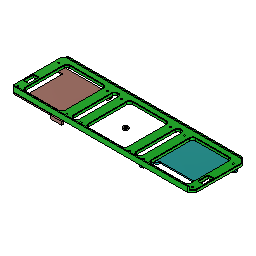
LCD sled v8 (Autodesk Fusion 360 design; units mm, degrees)
Autodesk Fusion 360 part; units mm, degrees
note: some values were not read from the file. Set by a fixed rule: which sketch regions a step uses; the direction of a hole.
sketch "Esquisse1" plane through (0, 0, 0) normal (0, 0, 1) x (1, 0, 0)
  circle A0 centre (107.25, 0) radius 1.25
  line L0 (136, 89.05) -> (136, -3.55)
  line L1 (136, -3.55) -> (-121, -3.55)
  line L2 (-121, -3.55) -> (-121, 89.05)
  line L3 (-121, 89.05) -> (136, 89.05)
  line L4 (108.5, 10.5227) -> (108.5, -1.25) construction
  line L5 (-112.6, 59.85) -> (117.25, 59.85)
  line L6 (117.25, 59.85) -> (117.25, -4.15)
  line L7 (117.25, -4.15) -> (-112.6, -4.15)
  line L8 (-112.6, -4.15) -> (-112.6, 59.85)
  line L9 (108.5, -1.25) -> (-108.5, -1.25) construction
  line L10 (-108.5, -1.25) -> (-108.5, 4.7567) construction
  circle A1 centre (-107.25, 0) radius 1.25
  circle A2 centre (-47.25, 0) radius 1.25
  circle A3 centre (-30, 0) radius 1.25
  circle A4 centre (30, 0) radius 1.25
  circle A5 centre (47.25, 0) radius 1.25
  point P0 (-107.25, 50)
  point P1 (-47.25, 50)
  point P2 (-30, 50)
  point P3 (30, 50)
  point P4 (47.25, 50)
  point P5 (107.25, 50)
  dimension "d1" = 27.5
  dimension "d2" = 8.75
  dimension "d3" = 2.5
  dimension "d4" = 12.5
  dimension "d5" = 5.35
  dimension "d6" = 0.6
  dimension "d7" = 2.3
  dimension "d8" = 60
  dimension "d9" = 60
  dimension "d10" = 60
  dimension "d11" = 17.25
  dimension "d12" = 17.25
  dimension "d13" = 30
  dimension "d14" = 92.6
  dimension "d15" = 64
  dimension "d16" = 50
  constraint vertical L0
  constraint perpendicular L0 L1
  constraint perpendicular L1 L2
  constraint horizontal L3
  constraint vertical L4
  constraint horizontal L5
  constraint vertical L6
  constraint horizontal L7
  constraint vertical L8
  constraint tangent A0 L4
  constraint perpendicular L8 L9
  constraint perpendicular L9 L10
  constraint equal A0 A1
  constraint horizontal origin A0.centre
  constraint horizontal origin A1.centre
  constraint tangent A0 L9
  constraint tangent L10 A1
  constraint equal A1 A2
  constraint tangent L9 A2
  constraint equal A4 A5
  constraint equal A3 A4
  constraint equal A2 A3
  constraint tangent L9 A3
  constraint tangent L9 A4
  constraint tangent L9 A5
  constraint horizontal P4 P5
  constraint horizontal P3 P4
  constraint horizontal P1 P2
  constraint horizontal P0 P1
  constraint vertical A1.centre P0
  constraint vertical A2.centre P1
  constraint vertical A3.centre P2
  constraint vertical A5.centre P4
  constraint vertical A0.centre P5
  constraint vertical A4.centre P3
  constraint horizontal P2 P3
  measures "d1" distance of L0 L4
  measures "d2" distance of L4 L6
  measures "d3" diameter of A0
  measures "d4" distance of L2 L10
  measures "d5" distance of L8 A1.centre
  measures "d6" distance of L1 L7
  measures "d7" distance of L1 L9
  measures "d8" distance of A1.centre A2.centre
  measures "d9" distance of A3.centre A4.centre
  measures "d10" horizontal distance of A0.centre A5.centre
  measures "d11" distance of A4.centre A5.centre
  measures "d12" distance of A2.centre A3.centre
  measures "d13" distance of origin A4.centre
  measures "d14" distance of L0.start L0.end
  measures "d15" distance of L5.end L6.end
  measures "d16" vertical distance of A1.centre P0
ref_plane "Plan de construction1" through (0, 0, 10.5) normal (0, 0, 1) x (1, 0, 0)
sketch "Esquisse2" plane through (0, 0, 10.5) normal (0, 0, 1) x (1, 0, 0)
  line L0 (-112.6, 59.85) -> (117.25, 59.85)
  line L1 (117.25, 59.85) -> (117.25, -4.15)
  line L2 (117.25, -4.15) -> (-112.6, -4.15)
  line L3 (-112.6, -4.15) -> (-112.6, 59.85)
extrude "Extrusion1" add sketch "Esquisse2" against normal blind 6.5 makes body 1
sketch "Esquisse3" plane through (0, 0, 0) normal (1, 0, 0) x (0, 1, 0)
  line L0 (-4.15, 10.5) -> (59.85, 10.5)
  line L1 (59.85, 10.5) -> (59.85, 4)
  line L2 (59.85, 4) -> (-4.15, 4)
  line L3 (-4.15, 4) -> (-4.15, 10.5)
  line L4 (-4.35, 10.7) -> (60.05, 10.7)
  line L5 (60.05, 10.7) -> (60.05, 3.8)
  line L6 (60.05, 3.8) -> (-4.35, 3.8)
  line L7 (-4.35, 3.8) -> (-4.35, 10.7)
  line L8 (-4.35, 6.8) -> (-5.55, 6.8)
  line L9 (-5.55, 6.8) -> (-5.55, 0)
  line L10 (-5.55, 0) -> (61.25, 0)
  line L11 (61.25, 0) -> (61.25, 5.05)
  line L12 (61.25, 5.05) -> (60.05, 5.05)
  dimension "d20" = -0.2
  dimension "d21" = 1.2
  dimension "d22" = 1.2
  dimension "d61" = 3
  dimension "d62" = 1.25
  constraint perpendicular L7 L8
  constraint perpendicular L8 L9
  constraint perpendicular L9 L10
  constraint perpendicular L8 L11
  constraint perpendicular L5 L12
  constraint coincident L10 origin
  constraint coincident L5 L12.end
  constraint coincident L7 L8.start
  measures "d21" distance of L5 L11
  measures "d22" distance of L7 L9
  measures "d61" distance of L6 L8
  measures "d62" vertical distance of L5.end L11.end
extrude "Extrusion2" add sketch "Esquisse3" along normal mid plane 224 separate body contours L5 L6 L7 L8 L9 L10 L11 L12 makes body 2
hole "Perçage1" at (-107.25, 0, 0) at (-47.25, 0, 0) at (-30, 0, 0) at (-30, 50, 0) at (-47.25, 50, 0) at (-107.25, 50, 0) at (30, 50, 0) at (30, 0, 0) at (47.25, 0, 0) at (47.25, 50, 0) at (107.25, 50, 0) at (107.25, 0, 0) direction (0, 0, 1) diameter 2 depth 5 tip angle 180 countersink diameter 2.4 countersink angle 90 bodies 2
sketch "Esquisse4" plane through (0, 0, 0) normal (0, 0, -1) x (1, 0, 0)
  circle A0 centre (107.25, -50) radius 1.2
  circle A1 centre (47.25, 0) radius 1.2
  circle A2 centre (30, -50) radius 1.2
  circle A3 centre (-47.25, -50) radius 1.2
  circle A4 centre (-30, 0) radius 1.2
  circle A5 centre (-107.25, 0) radius 1.2
  circle A6 centre (-47.25, 0) radius 1.2
  circle A7 centre (-30, -50) radius 1.2
  circle A8 centre (-107.25, -50) radius 1.2
  circle A9 centre (30, 0) radius 1.2
  circle A10 centre (47.25, -50) radius 1.2
  circle A11 centre (107.25, 0) radius 1.2
  line L0 (-112, -61.25) -> (112, -61.25)
  line L1 (112, -61.25) -> (112, 5.55)
  line L2 (112, 5.55) -> (-112, 5.55)
  line L3 (-112, 5.55) -> (-112, -61.25)
  line L4 (-110.25, -10) -> (-104.25, -10)
  line L5 (-104.25, -10) -> (-104.25, -22)
  line L6 (-104.25, -22) -> (-110.25, -22)
  line L7 (-110.25, -22) -> (-110.25, -10)
  line L8 (117.25, 4.15) -> (-112.6, 4.15)
  line L9 (-107.25, 0) -> (-107.25, -10) construction
  line L10 (-3, -22) -> (3, -22)
  line L11 (3, -22) -> (3, -10)
  line L12 (3, -10) -> (-3, -10)
  line L13 (-3, -10) -> (-3, -22)
  line L14 (0, 0) -> (0, -10) construction
  line L15 (104.25, -22) -> (110.25, -22)
  line L16 (110.25, -22) -> (110.25, -10)
  line L17 (110.25, -10) -> (104.25, -10)
  line L18 (104.25, -10) -> (104.25, -22)
  line L19 (107.25, 0) -> (107.25, -10) construction
  dimension "d32" = 6
  dimension "d33" = 12
  dimension "d63" = 10
  constraint horizontal L4
  constraint vertical L5
  constraint horizontal L6
  constraint vertical L7
  constraint coincident A5.centre L9.start
  constraint midpoint L4 L9.end
  constraint vertical L9
  constraint horizontal L10
  constraint vertical L11
  constraint horizontal L12
  constraint vertical L13
  constraint coincident L14.start origin
  constraint midpoint L12 L14.end
  constraint vertical L14
  constraint collinear L6 L10
  constraint collinear L4 L12
  constraint equal L6 L10
  constraint horizontal L15
  constraint vertical L16
  constraint horizontal L17
  constraint vertical L18
  constraint coincident A11.centre L19.start
  constraint midpoint L17 L19.end
  constraint vertical L19
  constraint equal L10 L15
  constraint collinear L10 L15
  constraint collinear L12 L17
  measures "d32" distance of L4.start L4.end
  measures "d33" distance of L4.end L5.end
  measures "d63" distance of L4 A5.centre
extrude "Extrusion3" cut sketch "Esquisse4" against normal up to surface (3.8 mm away) contours L4 L5 L6 L7 | L10 L11 L12 L13 | L15 L16 L17 L18 bodies 2
ref_plane "Plan de construction2" through (0, 27.85, -1.6) normal (0, 0, -1) x (0, 1, 0)
sketch "Esquisse5" plane through (0, 27.05, -1.6) normal (0, 0, -1) x (1, 0, 0)
  circle A0 centre (47.25, -22.95) radius 1.5
  circle A1 centre (47.25, 16.55) radius 1
  circle A2 centre (97.25, -22.95) radius 1
  circle A3 centre (107.25, -22.95) radius 1.5
  circle A4 centre (47.25, 27.05) radius 1.5
  line L0 (99.75, -25.7) -> (44.75, -25.7)
  line L1 (44.75, -25.7) -> (44.75, 19.3)
  line L2 (44.75, 19.3) -> (99.75, 19.3)
  line L3 (99.75, 19.3) -> (99.75, -25.7)
  line L4 (107.25, -20.2) -> (97.25, -20.2)
  arc A5 (97.25, -20.2) -> (97.25, -25.7) centre (97.25, -22.95) ccw
  line L5 (97.25, -25.7) -> (107.25, -25.7)
  arc A6 (107.25, -25.7) -> (107.25, -20.2) centre (107.25, -22.95) ccw
  line L6 (107.25, -22.95) -> (97.25, -22.95) construction
  line L7 (44.75, 27.05) -> (44.75, 16.55)
  arc A7 (44.75, 16.55) -> (49.75, 16.55) centre (47.25, 16.55) ccw
  line L8 (49.75, 16.55) -> (49.75, 27.05)
  arc A8 (49.75, 27.05) -> (44.75, 27.05) centre (47.25, 27.05) ccw
  line L9 (47.25, 27.05) -> (47.25, 16.55) construction
  circle A9 centre (47.25, 16.55) radius 2.5
  circle A10 centre (97.25, -22.95) radius 2.5
  circle A11 centre (47.25, -22.95) radius 2.5
  circle A12 centre (97.25, 16.55) radius 2.5
  point P0 (47.25, -22.95)
  point P1 (47.25, 27.05)
  point P2 (107.25, -22.95)
  dimension "d42" = 3
  dimension "d43" = 50
  dimension "d44" = 39.5
  dimension "d45" = 2
  dimension "d46" = 55
  dimension "d48" = 45
  dimension "d49" = 2.75
  dimension "d50" = 2.5
  dimension "d51" = 2.75
  dimension "d52" = 2.5
  constraint coincident P0 A0.centre
  constraint coincident P1 A4.centre
  constraint coincident P2 A3.centre
  constraint equal A0 A3
  constraint equal A3 A4
  constraint equal A1 A2
  constraint horizontal L0
  constraint vertical L1
  constraint horizontal L2
  constraint vertical L3
  constraint vertical A1.centre P1
  constraint horizontal A2.centre P0
  constraint tangent L4 A5
  constraint tangent A5 L5
  constraint parallel L4 L5
  constraint tangent L5 A6
  constraint tangent L4 A6
  constraint coincident A2.centre A5.centre
  constraint horizontal L6
  constraint tangent L7 A7
  constraint tangent A7 L8
  constraint parallel L7 L8
  constraint tangent L8 A8
  constraint tangent L7 A8
  constraint coincident A1.centre A7.centre
  constraint perpendicular L2 L9
  constraint concentric A1 A9
  constraint equal A8 A9
  constraint concentric A5 A10
  constraint tangent L3 A10
  constraint equal A10 A11
  constraint equal A9 A12
  constraint horizontal A1.centre A12.centre
  constraint vertical A2.centre A12.centre
  measures "d42" diameter of A0
  measures "d43" horizontal distance of A2.centre P0
  measures "d44" vertical distance of A1.centre P0
  measures "d45" diameter of A2
  measures "d46" distance of L0.start L0.end
  measures "d48" distance of L0.end L1.end
  measures "d49" distance of A1.centre L2
  measures "d50" distance of A2.centre L3
  measures "d51" radius of A6
  measures "d52" radius of A8
extrude "Extrusion4" add sketch "Esquisse5" along normal blind 2 separate body contours A10 | L0 L3 L4 A5 L5 | L3 L4 L5 A6 | A12 | A11 | L0 L1 L2 L3 L4 A5 A7 L8 A9 | A7 A9 | L1 L2 L7 L8 A9 | L2 L7 L8 A8 makes body 3
extrude "Extrusion5" add sketch "Esquisse5" along normal blind 2 from surface at 2 contours A10 | A12 | A11 | A7 A9 bodies 3
fillet "Congé1" radius 2 4 edges at (99.75, 47.25, -2.6) (99.75, 7.75, -2.6) (49.75, 7.75, -2.6) (44.75, 52.75, -2.6) on bodies 3
chamfer "Chanfrein1" distance 0.5 angle 45 5 edges at (96.3177, 49.6384, -5.6) (46.3177, 10.1384, -5.6) (45.8515, 49.4576, -5.6) (45.8515, -0.5424, -3.6) (105.8515, 49.4576, -3.6) on bodies 3
sketch "Esquisse6" plane through (0, 0, 3.8) normal (0, 0, 1) x (-1, 0, 0)
  line L0 (110.25, -10) -> (110.25, -22)
  line L1 (110.25, -22) -> (104.25, -22)
  line L2 (104.25, -22) -> (104.25, -10)
  line L3 (104.25, -10) -> (110.25, -10)
  line L4 (-3, -10) -> (3, -10)
  line L5 (3, -10) -> (3, -22)
  line L6 (3, -22) -> (-3, -22)
  line L7 (-3, -22) -> (-3, -10)
  line L8 (-110.25, -10) -> (-104.25, -10)
  line L9 (-104.25, -10) -> (-104.25, -22)
  line L10 (-104.25, -22) -> (-110.25, -22)
  line L11 (-110.25, -22) -> (-110.25, -10)
  circle A0 centre (-107.25, -50) radius 1
  circle A1 centre (-47.25, 0) radius 1
  circle A2 centre (-30, -50) radius 1
  circle A3 centre (47.25, -50) radius 1
  circle A4 centre (30, 0) radius 1
  circle A5 centre (107.25, 0) radius 1
  circle A6 centre (47.25, 0) radius 1
  circle A7 centre (30, -50) radius 1
  circle A8 centre (107.25, -50) radius 1
  circle A9 centre (-30, 0) radius 1
  circle A10 centre (-47.25, -50) radius 1
  circle A11 centre (-107.25, 0) radius 1
  line L12 (112, 4.35) -> (-112, 4.35)
  line L13 (-112, 4.35) -> (-112, -60.05)
  line L14 (-112, -60.05) -> (112, -60.05)
  line L15 (112, -60.05) -> (112, 4.35)
  line L16 (101.25, -54.05) -> (53.25, -54.05)
  line L17 (53.25, -54.05) -> (53.25, 0)
  line L18 (53.25, 0) -> (101.25, 0)
  line L19 (101.25, 0) -> (101.25, -54.05)
  line L20 (42.25, -54.05) -> (35, -54.05)
  line L21 (35, -54.05) -> (35, 0)
  line L22 (35, 0) -> (42.25, 0)
  line L23 (42.25, 0) -> (42.25, -54.05)
  line L24 (24, -54.05) -> (-24, -54.05)
  line L25 (-24, -54.05) -> (-24, 0)
  line L26 (-24, 0) -> (24, 0)
  line L27 (24, 0) -> (24, -54.05)
  line L28 (-53.25, -54.05) -> (-101.25, -54.05)
  line L29 (-101.25, -54.05) -> (-101.25, 0)
  line L30 (-101.25, 0) -> (-53.25, 0)
  line L31 (-53.25, 0) -> (-53.25, -54.05)
  line L32 (-35, -54.05) -> (-42.25, -54.05)
  line L33 (-42.25, -54.05) -> (-42.25, 0)
  line L34 (-42.25, 0) -> (-35, 0)
  line L35 (-35, 0) -> (-35, -54.05)
  dimension "d64" = 6
  dimension "d65" = 6
  dimension "d66" = 6
  dimension "d67" = 5
  dimension "d68" = 5
  dimension "d69" = 6
  dimension "d70" = 6
  dimension "d71" = 5
  constraint horizontal L16
  constraint vertical L17
  constraint horizontal L18
  constraint vertical L19
  constraint coincident A5.centre L18
  constraint horizontal L20
  constraint vertical L21
  constraint horizontal L22
  constraint vertical L23
  constraint horizontal L24
  constraint vertical L25
  constraint horizontal L26
  constraint vertical L27
  constraint horizontal L28
  constraint vertical L29
  constraint horizontal L30
  constraint vertical L31
  constraint collinear L26 L30
  constraint collinear L18 L26
  constraint collinear L24 L28
  constraint collinear L16 L20
  constraint collinear L22 L26
  constraint collinear L20 L24
  constraint equal L24 L28
  constraint equal L16 L28
  constraint horizontal L32
  constraint vertical L33
  constraint horizontal L34
  constraint vertical L35
  constraint equal L20 L32
  constraint collinear L28 L32
  constraint collinear L30 L34
  measures "d64" distance of A3.centre L17
  measures "d65" distance of A8.centre L19
  measures "d66" distance of L14 L16
  measures "d67" distance of A6.centre L23
  measures "d68" distance of A4.centre L21
  measures "d69" distance of A2.centre L25
  measures "d70" distance of A10.centre L31
  measures "d71" distance of A10.centre L33
extrude "Extrusion6" cut sketch "Esquisse6" against normal up to surface (3.8 mm away) contours L16 L17 L18 L19 | L20 L21 L22 L23 | L24 L25 L26 L27 | L28 L29 L30 L31 | L32 L33 L34 L35 bodies 2
fillet "Congé2" radius 3.5 20 edges at (24, 54.05, 1.9) (42.25, 54.05, 1.9) (101.25, 54.05, 1.9) (-35, 54.05, 1.9) (-53.25, 54.05, 1.9) (53.25, 54.05, 1.9) (35, 54.05, 1.9) (-24, 54.05, 1.9) (-42.25, 54.05, 1.9) (-101.25, 54.05, 1.9) (-35, 0, 1.9) (-53.25, 0, 1.9) (-101.25, 0, 1.9) (-42.25, 0, 1.9) (-24, 0, 1.9) (24, 0, 1.9) (35, 0, 1.9) (42.25, 0, 1.9) (53.25, 0, 1.9) (101.25, 0, 1.9) on bodies 2
chamfer "Chanfrein2" distance 5 angle 45 4 edges at (112, 61.25, 2.525) (112, -5.55, 3.4) (-112, -5.55, 3.4) (-112, 61.25, 2.525) on bodies 2
chamfer "Chanfrein3" distance 0.5 angle 45 114 edges at (-77.25, 54.05, 3.8) (-54.2751, 53.0249, 3.8) (-53.25, 27.025, 3.8) (-54.2751, 1.0251, 3.8) (-77.25, 0, 3.8) (-100.2249, 1.0251, 3.8) (-101.25, 27.025, 3.8) (-100.2249, 53.0249, 3.8) (0, 54.05, 3.8) (22.9749, 53.0249, 3.8) (24, 27.025, 3.8) (22.9749, 1.0251, 3.8) (0, 0, 3.8) (-22.9749, 1.0251, 3.8) (-24, 27.025, 3.8) (-22.9749, 53.0249, 3.8) (-36.0251, 53.0249, 3.8) (-38.625, 54.05, 3.8) (-41.2249, 53.0249, 3.8) (-42.25, 27.025, 3.8) (-41.2249, 1.0251, 3.8) (-38.625, 0, 3.8) (-36.0251, 1.0251, 3.8) (-35, 27.025, 3.8) (-110.1, -2.45, 3.8) (-112, 27.85, 3.8) (-110.1, 58.15, 3.8) (-104.25, 16, 3.8) (-107.25, 22, 3.8) (-107.25, 10, 3.8) (-110.25, 16, 3.8) (35, 27.025, 3.8) (36.0251, 53.0249, 3.8) (38.625, 54.05, 3.8) (41.2249, 53.0249, 3.8) (42.25, 27.025, 3.8) (41.2249, 1.0251, 3.8) (38.625, 0, 3.8) (36.0251, 1.0251, 3.8) (53.25, 27.025, 3.8) (54.2751, 53.0249, 3.8) (77.25, 54.05, 3.8) (100.2249, 53.0249, 3.8) (101.25, 27.025, 3.8) (100.2249, 1.0251, 3.8) (77.25, 0, 3.8) (54.2751, 1.0251, 3.8) (104.25, 16, 3.8) (107.25, 22, 3.8) (110.25, 16, 3.8) (107.25, 10, 3.8) (112, 27.85, 3.8) (110.1, -2.45, 3.8) (110.1, 58.15, 3.8) (108.2, -4.35, 5.3) (108.2, 60.05, 4.425) (-108.2, 60.05, 4.425) (-108.2, -4.35, 5.3) (-24, 27.025, 0) (-22.9749, 1.0251, 0) (0, 0, 0) (22.9749, 1.0251, 0) (24, 27.025, 0) (22.9749, 53.0249, 0) (0, 54.05, 0) (-22.9749, 53.0249, 0) (-35, 27.025, 0) (-36.0251, 53.0249, 0) (-38.625, 54.05, 0) (-41.2249, 53.0249, 0) (-42.25, 27.025, 0) (-41.2249, 1.0251, 0) (-38.625, 0, 0) (-36.0251, 1.0251, 0) (-53.25, 27.025, 0) (-54.2751, 53.0249, 0) (-77.25, 54.05, 0) (-100.2249, 53.0249, 0) (-101.25, 27.025, 0) (-100.2249, 1.0251, 0) (-77.25, 0, 0) (-54.2751, 1.0251, 0) (35, 27.025, 0) (36.0251, 1.0251, 0) (38.625, 0, 0) (41.2249, 1.0251, 0) (42.25, 27.025, 0) (41.2249, 53.0249, 0) (38.625, 54.05, 0) (36.0251, 53.0249, 0) (101.25, 27.025, 0) (100.2249, 53.0249, 0) (77.25, 54.05, 0) (54.2751, 53.0249, 0) (53.25, 27.025, 0) (54.2751, 1.0251, 0) (77.25, 0, 0) (100.2249, 1.0251, 0) (0, -5.55, 0) (109.5, -3.05, 0) (112, 27.85, 0) (109.5, 58.75, 0) (0, 61.25, 0) (107.25, 22, 0) (104.25, 16, 0) (107.25, 10, 0) (110.25, 16, 0) (-109.5, -3.05, 0) (-112, 27.85, 0) (-109.5, 58.75, 0) (-107.25, 22, 0) (-110.25, 16, 0) (-107.25, 10, 0) (-104.25, 16, 0) on bodies 2
sketch "Esquisse7" plane through (0, 0, 0) normal (0, 0, 1) x (1, 0, 0)
  circle A0 centre (0.258, 24.8864) radius 3
  circle A1 centre (0.258, 24.8864) radius 1.6
  dimension "d78" = 3.2
  dimension "d79" = 6
  constraint concentric A0 A1
  measures "d78" diameter of A1
  measures "d79" diameter of A0
extrude "Extrusion7" add sketch "Esquisse7" along normal blind 1.5 separate body makes body 4
sketch "Esquisse8" plane through (0, 27.85, -1.6) normal (0, 0, -1) x (1, 0, 0)
  circle A0 centre (47.25, -28.15) radius 2.5
  circle A1 centre (97.25, -28.15) radius 2.5
  circle A2 centre (47.25, 11.35) radius 2.5
  circle A3 centre (97.25, 11.35) radius 2.5
  line L0 (101.25, -32.15) -> (43.25, -32.15)
  line L1 (43.25, -32.15) -> (43.25, 15.35)
  line L2 (43.25, 15.35) -> (101.25, 15.35)
  line L3 (101.25, 15.35) -> (101.25, -32.15)
  circle A4 centre (47.25, -22.15) radius 1.5
  line L4 (43.25, 27.85) -> (43.25, 11.35)
  arc A5 (43.25, 11.35) -> (51.25, 11.35) centre (47.25, 11.35) ccw
  line L5 (51.25, 11.35) -> (51.25, 27.85)
  arc A6 (51.25, 27.85) -> (43.25, 27.85) centre (47.25, 27.85) ccw
  line L6 (47.25, 27.85) -> (47.25, 11.35) construction
  circle A7 centre (47.25, 27.85) radius 1.5
  circle A8 centre (47.25, 27.85) radius 1
  circle A9 centre (107.25, -22.15) radius 1.5
  line L7 (105.192, -18.72) -> (95.192, -24.72)
  arc A10 (95.192, -24.72) -> (99.308, -31.58) centre (97.25, -28.15) ccw
  line L8 (99.308, -31.58) -> (109.308, -25.58)
  arc A11 (109.308, -25.58) -> (105.192, -18.72) centre (107.25, -22.15) ccw
  line L9 (107.25, -22.15) -> (97.25, -28.15) construction
  circle A12 centre (107.25, -22.15) radius 1.2
  point P0 (47.25, -22.15)
  dimension "d82" = 50
  dimension "d83" = 39.5
  dimension "d84" = 5
  dimension "d85" = 6
  dimension "d86" = 4
  dimension "d87" = 4
  dimension "d88" = 4
  dimension "d89" = 4
  dimension "d90" = 3
  dimension "d91" = 3
  constraint horizontal A0.centre A1.centre
  constraint vertical A0.centre A2.centre
  constraint horizontal A2.centre A3.centre
  constraint vertical A1.centre A3.centre
  constraint equal A0 A2
  constraint equal A2 A3
  constraint equal A1 A3
  constraint vertical A0.centre P0
  constraint horizontal L0
  constraint vertical L1
  constraint horizontal L2
  constraint vertical L3
  constraint coincident P0 A4.centre
  constraint tangent L4 A5
  constraint tangent A5 L5
  constraint parallel L4 L5
  constraint tangent L5 A6
  constraint tangent L4 A6
  constraint coincident A2.centre A5.centre
  constraint coincident A6.centre L6.start
  constraint concentric A7 A8
  constraint collinear L1 L4
  constraint equal A7 A9
  constraint tangent L7 A10
  constraint tangent A10 L8
  constraint parallel L7 L8
  constraint tangent L8 A11
  constraint tangent L7 A11
  constraint coincident A1.centre A10.centre
  constraint coincident A9.centre A11.centre
  constraint equal A5 A10
  constraint concentric A9 A12
  measures "d82" distance of A0.centre A1.centre
  measures "d83" distance of A0.centre A2.centre
  measures "d84" diameter of A0
  measures "d85" vertical distance of A0.centre P0
  measures "d86" distance of A2.centre L1
  measures "d87" distance of A2.centre L2
  measures "d88" distance of A1.centre L3
  measures "d89" distance of A0.centre L0
  measures "d90" diameter of A4
  measures "d91" diameter of A7
extrude "Extrusion8" add sketch "Esquisse8" along normal blind 1.5 separate body contours A0 | A1 | A2 | A3 | L0 L1 L2 L3 A5 L5 L7 A10 | L3 L7 A10 L8 | L3 L7 L8 A11 | L1 L2 L4 A5 L5 | L2 L4 L5 A6 makes body 5
extrude "Extrusion9" add sketch "Esquisse8" along normal blind 7 contours A0 | A1 | A2 | A3 bodies 5
hole "Perçage2" at (97.25, 56, -1.6) at (97.25, 16.5, -1.6) at (47.25, 16.5, -1.6) at (47.25, 56, -1.6) direction (0, 0, -1) diameter 2 depth 10 tip angle 118 bodies 5
fillet "Congé3" radius 3.5 4 edges at (101.25, 12.5, -2.35) (43.25, 60, -2.35) (51.25, 12.5, -2.35) (101.25, 48.9352, -2.35) on bodies 5
fillet "Congé4" radius 1 4 edges at (94.9192, 55.096, -3.1) (94.9192, 15.596, -3.1) (44.9192, 15.596, -3.1) (44.9192, 55.096, -3.1) on bodies 5
sketch "Esquisse9" plane through (0, 0, -1.6) normal (0, 0, 1) x (-1, 0, 0)
  circle A0 centre (-47.25, -16.5) radius 1
  circle A1 centre (-97.25, -56) radius 1
  circle A2 centre (-97.25, -16.5) radius 1
  circle A3 centre (-47.25, -56) radius 1
  circle A4 centre (-107.25, -50) radius 1.5
  circle A5 centre (-47.25, 0) radius 1.5
  circle A6 centre (-47.25, -50) radius 1.5
  arc A7 (-46.75, -60) -> (-43.25, -56.5) centre (-46.75, -56.5) ccw
  line L0 (-43.25, -56.5) -> (-43.25, 0)
  arc A8 (-43.25, 0) -> (-51.25, 0) centre (-47.25, 0) ccw
  line L1 (-51.25, 0) -> (-51.25, -9)
  arc A9 (-54.75, -12.5) -> (-51.25, -9) centre (-54.75, -9) ccw
  line L2 (-54.75, -12.5) -> (-97.75, -12.5)
  arc A10 (-97.75, -12.5) -> (-101.25, -16) centre (-97.75, -16) ccw
  line L3 (-101.25, -16) -> (-101.25, -42.9289)
  arc A11 (-105.9167, -46.2288) -> (-101.25, -42.9289) centre (-104.75, -42.9289) ccw
  arc A12 (-105.9167, -46.2288) -> (-109.308, -53.43) centre (-107.25, -50) ccw
  line L4 (-109.308, -53.43) -> (-99.308, -59.43)
  arc A13 (-99.308, -59.43) -> (-97.25, -60) centre (-97.25, -56) ccw
  line L5 (-97.25, -60) -> (-46.75, -60)
  line L6 (47.25, -54) -> (107.25, -54)
  arc A14 (107.25, -54) -> (107.25, -46) centre (107.25, -50) ccw
  line L7 (107.25, -46) -> (47.25, -46)
  arc A15 (47.25, -46) -> (47.25, -54) centre (47.25, -50) ccw
  line L8 (47.25, -50) -> (107.25, -50) construction
  circle A16 centre (47.25, -50) radius 1.2
  circle A17 centre (107.25, -50) radius 1.2
  line L9 (47.25, -4) -> (107.25, -4)
  arc A18 (107.25, -4) -> (107.25, 4) centre (107.25, 0) ccw
  line L10 (107.25, 4) -> (47.25, 4)
  arc A19 (47.25, 4) -> (47.25, -4) centre (47.25, 0) ccw
  line L11 (47.25, 0) -> (107.25, 0) construction
  circle A20 centre (47.25, 0) radius 1.2
  line L12 (98.25, -46) -> (48.25, -46)
  line L13 (48.25, -46) -> (48.25, -4)
  line L14 (48.25, -4) -> (98.25, -4)
  line L15 (98.25, -4) -> (98.25, -46)
  line L16 (98.25, -46) -> (48.25, -4) construction
  line L17 (48.25, -46) -> (98.25, -4) construction
  line L18 (48.25, -4) -> (48.25, 4)
  point P0 (73.25, -25)
  point P1 (77.25, -54)
  dimension "d103" = 4
  dimension "d104" = 50
  dimension "d105" = 4
  constraint tangent L6 A14
  constraint tangent A14 L7
  constraint parallel L6 L7
  constraint tangent L7 A15
  constraint tangent L6 A15
  constraint concentric A15 A16
  constraint concentric A14 A17
  constraint tangent L9 A18
  constraint tangent A18 L10
  constraint parallel L9 L10
  constraint tangent L10 A19
  constraint tangent L9 A19
  constraint horizontal L11
  constraint equal A15 A19
  constraint equal L8 L11
  constraint concentric A19 A20
  constraint horizontal L12
  constraint perpendicular L12 L13
  constraint parallel L12 L14
  constraint parallel L13 L15
  constraint coincident L16 P0
  constraint coincident L17 P0
  constraint collinear L7 L12
  constraint collinear L9 L14
  constraint coincident L6 P1
  constraint midpoint L6 P1
  constraint coincident L10 L18.end
  constraint perpendicular L10 L18
  measures "d103" radius of A15
  measures "d104" distance of L13 L15
  measures "d105" horizontal distance of P0 P1
extrude "Extrusion10" add sketch "Esquisse9" against normal up to surface (1.5 mm away) separate body contours L6 A14 L7 A15 L12 | L7 L9 L12 L13 L14 L15 | L9 A18 L10 A20 L14 L18 | A20 L18 | A16 | A17 picked at (48.2787, -0.1701) makes body 6
hole "Perçage3" at (-47.25, 50, -1.6) at (-107.25, 50, -1.6) at (-107.25, 0, -1.6) direction (0, 0, -1) diameter 3.4 depth 20 tip angle 118 bodies 6
sketch "Esquisse10" plane through (0, 0, -3.1) normal (0, 0, -1) x (1, 0, 0)
  circle A0 centre (-47.25, -50) radius 1.7
  circle A1 centre (-107.25, -50) radius 1.7
  circle A2 centre (-107.25, 0) radius 1.7
  line L0 (-48.25, 4) -> (-107.25, 4)
  arc A3 (-107.25, 4) -> (-107.25, -4) centre (-107.25, 0) ccw
  line L1 (-107.25, -4) -> (-98.25, -4)
  line L2 (-98.25, -4) -> (-98.25, -46)
  line L3 (-98.25, -46) -> (-107.25, -46)
  arc A4 (-107.25, -46) -> (-107.25, -54) centre (-107.25, -50) ccw
  line L4 (-107.25, -54) -> (-47.25, -54)
  arc A5 (-47.25, -54) -> (-47.25, -46) centre (-47.25, -50) ccw
  line L5 (-47.25, -46) -> (-48.25, -46)
  line L6 (-48.25, -46) -> (-48.25, 4)
  line L7 (-47, -43.6) -> (-89.25, -43.6)
  line L8 (-89.25, -43.6) -> (-89.25, -28.5)
  line L9 (-89.25, -28.5) -> (-47, -28.5)
  line L10 (-47, -28.5) -> (-47, -43.6)
  line L11 (-54.1, -43.6) -> (-67.7, -43.6)
  line L12 (-67.7, -43.6) -> (-67.7, -35.25)
  line L13 (-67.7, -35.25) -> (-54.1, -35.25)
  line L14 (-54.1, -35.25) -> (-54.1, -43.6)
  line L15 (-71.8, -43.6) -> (-85.4, -43.6)
  line L16 (-85.4, -43.6) -> (-85.4, -35.25)
  line L17 (-85.4, -35.25) -> (-71.8, -35.25)
  line L18 (-71.8, -35.25) -> (-71.8, -43.6)
  line L19 (-91.25, -26.5) -> (-45, -26.5)
  line L20 (-45, -26.5) -> (-45, -45.6)
  line L21 (-45, -45.6) -> (-91.25, -45.6)
  line L22 (-91.25, -45.6) -> (-91.25, -26.5)
  line L23 (-89.25, -26.5) -> (-56.25, -26.5)
  line L24 (-56.25, -26.5) -> (-56.25, -8.15)
  line L25 (-56.25, -8.15) -> (-89.25, -8.15)
  line L26 (-89.25, -8.15) -> (-89.25, -26.5)
  line L27 (-54.25, -28.5) -> (-54.25, -6.15)
  line L28 (-54.25, -6.15) -> (-91.25, -6.15)
  line L29 (-91.25, -6.15) -> (-91.25, -28.5)
  line L30 (-91.25, -28.5) -> (-54.25, -28.5)
  line L31 (-48.25, -6.15) -> (-60.25, -6.15)
  line L32 (-60.25, -6.15) -> (-60.25, 3.4)
  line L33 (-60.25, 3.4) -> (-48.25, 3.4)
  line L34 (-48.25, 3.4) -> (-48.25, -6.15)
  line L35 (-46.25, 5.4) -> (-46.25, -8.15)
  line L36 (-46.25, -8.15) -> (-62.25, -8.15)
  line L37 (-62.25, -8.15) -> (-62.25, 5.4)
  line L38 (-62.25, 5.4) -> (-46.25, 5.4)
  line L39 (-48.25, 3.4) -> (-48.25, 5.4)
  dimension "d111" = 42.25
  dimension "d112" = 13.6
  dimension "d113" = 4.1
  dimension "d114" = 7.1
  dimension "d115" = 15.1
  dimension "d116" = 6.75
  dimension "d117" = -2
  dimension "d118" = 7
  dimension "d119" = 30.5
  dimension "d123" = 18.35
  dimension "d124" = 33
  dimension "d125" = 2
  dimension "d126" = 12
  dimension "d127" = 9.55
  dimension "d128" = -2
  constraint horizontal L7
  constraint vertical L8
  constraint horizontal L9
  constraint vertical L10
  constraint horizontal L11
  constraint vertical L12
  constraint horizontal L13
  constraint vertical L14
  constraint coincident L7 L11.start
  constraint horizontal L15
  constraint vertical L16
  constraint horizontal L17
  constraint vertical L18
  constraint coincident L7 L15.start
  constraint equal L13 L17
  constraint equal L12 L18
  constraint horizontal L23
  constraint vertical L24
  constraint horizontal L25
  constraint vertical L26
  constraint coincident L19 L23.start
  constraint collinear L8 L26
  constraint horizontal L31
  constraint vertical L32
  constraint horizontal L33
  constraint vertical L34
  constraint collinear L6 L34
  constraint collinear L28 L31
  constraint coincident L38 L39.end
  constraint perpendicular L38 L39
  measures "d111" distance of L8.end L9.end
  measures "d112" distance of L12.end L13.end
  measures "d113" distance of L12 L18
  measures "d114" distance of L10 L14
  measures "d115" distance of L7.end L8.end
  measures "d116" distance of L9 L17
  measures "d118" distance of L2 L22
  measures "d119" distance of L0 L19
  measures "d123" distance of L23.start L25.end
  measures "d124" distance of L24.end L25.end
  measures "d126" distance of L32.end L33.end
  measures "d127" distance of L31.end L32.end
extrude "Extrusion12" add sketch "Esquisse10" against normal up to surface (1.5 mm away) contours L0 L37 L38 L39 bodies 6
extrude "Extrusion11" add sketch "Esquisse10" along normal blind 3 contours L0 L6 L28 L32 L33 L37 L39 | L0 L37 L38 L39 | L19 L25 L26 L28 L29 L37 | L25 L27 L28 L31 L36 L37 | L6 L27 L31 L36 | L9 L19 L22 L23 L27 L29 L30 | L19 L24 L27 L36 | L6 L9 L19 L27 | L6 L7 L8 L11 L15 L21 L22 L30 | L7 L11 L12 L13 L14 | L7 L15 L16 L17 L18 bodies 6
chamfer "Chanfrein4" distance 0.5 angle 45 1 faces at (-63.1667, 38.0333, -6.1) on bodies 6
hidden bodies 1 3
equation "d9 = d8"
equation "d10 = d9"
equation "d12 = d11"
equation "d13 = d9 / 2"
equation "d49 = ( d48 - d44 ) / 2"
equation "d50 = ( d46 - d43 ) / 2"
equation "d64 = d65"
equation "d68 = d67"
equation "d69 = d64"
equation "d70 = d69"
equation "d71 = d68"
equation "d87 = d86"
equation "d88 = d86"
equation "d89 = d86"
named bodies: "LCD", "LCD Sled", "LCD Controller holder", "LCD washer", "LCD Controller holder v2", "LCD Electronics holder"
